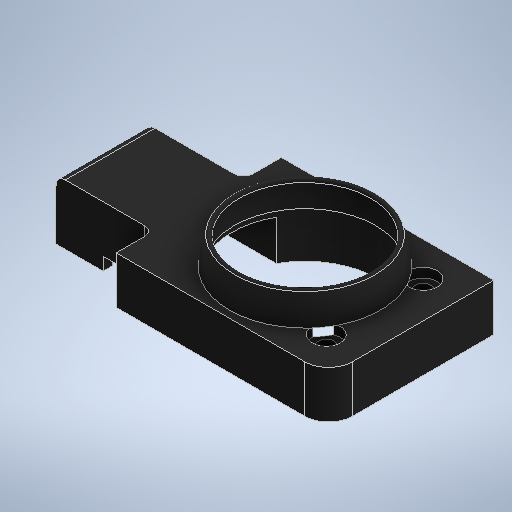
# Autodesk Inventor part: Joystick Shield
Saved by Autodesk Inventor 2025.4 (Build 294407000, 407)
## iProperties
Created: 2026-03-20
Part Number: Joystick Shield
Material: Generic
Document SubType Name: Modeling
Designer: lenovo
Density: 1 g/cm^3
Appearance: Default(1)
Author: lenovo
Autodesk Inventor part; units mm, degrees
ref_plane "YZ Plane" through (0, 0, 0) normal (1, 0, 0) x (0, 1, 0)
ref_plane "XZ Plane" through (0, 0, 0) normal (0, 1, 0) x (-1, 0, 0)
ref_plane "XY Plane" through (0, 0, 0) normal (0, 0, 1) x (1, 0, 0)
sketch "Sketch1" plane through (0, 0, 0) normal (0, 0, 1) x (1, 0, 0)
  line L0 (-22.5, -5) -> (22.5, -5)
  line L1 (22.5, -5) -> (22.5, 5)
  line L2 (22.5, 5) -> (-22.5, 5)
  line L3 (-22.5, 5) -> (-22.5, -5)
  line L4 (-22.5, -5) -> (22.5, 5) construction
  line L5 (22.5, -5) -> (-22.5, 5) construction
  point P0 (0, 0)
  dimension "d0" = 45
  dimension "d1" = 10
  constraints: 12 end point, 2 midpoint, 2 parallel, 1 horizontal, 1 perpendicular
  measures "d0" distance of L2.end L1.end
  measures "d1" distance of L2.end L0.start
extrude "Extrusion1" add sketch "Sketch1" along normal mid plane 35
sketch "Sketch2" plane through (0, 0, 0) normal (0, 0, 1) x (1, 0, 0)
  arc A0 (15, 5) -> (13.65, 11.2191) centre (0, 5) ccw
  line L0 (22.5, 5) -> (-22.5, 5) projected
  arc A1 (16, 5) -> (14.7419, 11.2191) centre (0, 5) ccw
  line L1 (13.65, 11.2191) -> (14.7419, 11.2191)
  line L2 (-22.5, -5) -> (22.5, -5) projected
  line L3 (0, -5) -> (0, 5)
  point P0 (0, 0)
  dimension "d4" = 15
  dimension "d6" = 1
  dimension "d24" = 27.3
  constraints: 4 end point, 4 point on circle, 3 midpoint, 2 centre point, 2 point on line, 1 coincident, 1 horizontal, 1 perpendicular
  measures "d4" radius of A0
  measures "d6" radial gap between concentric circles of A0 A1
  measures "d24" diameter of L1.start L3
revolve "Revolution1" add sketch "Sketch2" angle 360 about axis through (0, -5, 0) along (0, 1, 0)
fillet "Fillet1" radius 0.5 2 edges at (-14.7419, 11.2191, 0) (-13.65, 11.2191, 0)
sketch "Sketch3" plane through (-22.5, -5, 17.5) normal (0, -1, 0) x (1, 0, 0)
  circle A0 centre (22.5, -17.5) radius 14.75
  line L0 (45, 0) -> (45, -35) projected
  line L1 (0, 0) -> (45, 0) projected
  circle A1 centre (22.5, -17.5) radius 15 projected
  point P0 (45, -17.5)
  point P1 (22.5, 0)
  dimension "d9" = 29.5
  constraints: 2 midpoint, 1 centre point, 1 coincident, 1 concentric
  measures "d9" diameter of A0
extrude "Extrusion2" cut sketch "Sketch3" against normal up to surface (10 mm away) contours A0
sketch "Sketch4" plane through (-22.5, 5, 17.5) normal (0, 1, 0) x (1, 0, 0)
  circle A0 centre (37.25, 27.75) radius 1.65
  line L0 (45, 35) -> (45, 0) projected
  line L1 (0, 35) -> (45, 35) projected
  point P0 (22.5, 17.5)
  dimension "d12" = 3.3
  dimension "d13" = 7.75
  dimension "d14" = 7.25
  constraints: 1 centre point
  measures "d12" diameter of A0
  measures "d13" distance from line of L0 A0.centre
  measures "d14" distance from line of L1 A0.centre
extrude "Extrusion3" cut sketch "Sketch4" against normal blind 10
pattern_linear "Rectangular Pattern1" count 2 spacing 20.5 along (0, 0, 1) of "Extrusion3"
sketch "Sketch6" plane through (-22.5, -5, 17.5) normal (-1, 0, 0) x (0, 0, 1)
  line L0 (-10, 0) -> (-25, 0)
  line L1 (-25, 0) -> (-25, 8.5)
  line L2 (-25, 8.5) -> (-10, 8.5)
  line L3 (-10, 8.5) -> (-10, 0)
  line L4 (-10, 0) -> (-25, 8.5) construction
  line L5 (-25, 0) -> (-10, 8.5) construction
  line L6 (-35, 10) -> (0, 10) projected
  line L7 (0, 10) -> (0, 0) projected
  line L8 (-35, 0) -> (0, 0) projected
  point P0 (-17.5, 5)
  point P1 (-17.5, 4.25)
  point P2 (-17.5, 10)
  point P3 (-17.5, 0)
  dimension "d33" = 1.5
  dimension "d38" = 15
  constraints: 12 end point, 5 midpoint, 2 parallel, 1 horizontal, 1 perpendicular, 1 vertical alignment
  measures "d33" distance between parallel lines of L2 L6
  measures "d38" distance of L0.start L0.end
extrude "Extrusion5" cut sketch "Sketch6" against normal blind 15
sketch "Sketch8" plane through (-22.5, -5, -17.5) normal (0, -1, 0) x (1, 0, 0)
  circle A0 centre (22.5, 17.5) radius 15.5
  arc A1 (9.7991, 10) -> (9.7991, 25) centre (22.5, 17.5) ccw projected
  dimension "d39" = 31
  constraints: 1 centre point, 1 concentric
  measures "d39" diameter of A0
extrude "Extrusion6" cut sketch "Sketch8" against normal up to surface (10 mm away)
sketch "Sketch10" plane through (0, 0, 0) normal (0, 0, 1) x (1, 0, 0)
  line L0 (-22.5, -0.75) -> (-37.5, -0.75)
  line L1 (-37.5, -0.75) -> (-37.5, -7.75)
  line L2 (-22.5, 3.5) -> (-22.5, -5) projected
  point P0 (0, 0)
  dimension "d42" = 15
  dimension "d43" = 7
  constraints: 4 end point, 1 horizontal, 1 midpoint, 1 perpendicular
  measures "d42" distance of L0.start L0.end
  measures "d43" distance of L0.end L1.end
sketch "Sketch11" plane through (-22.5, -5, 17.5) normal (-1, 0, 0) x (0, 0, 1)
  line L0 (-27, 0) -> (-8, 0)
  line L1 (-8, 0) -> (-8, 10)
  line L2 (-8, 10) -> (-27, 10)
  line L3 (-27, 10) -> (-27, 0)
  line L4 (-27, 0) -> (-8, 10) construction
  line L5 (-8, 0) -> (-27, 10) construction
  line L6 (-35, 10) -> (0, 10) projected
  line L7 (-25, 8.5) -> (-10, 8.5) projected
  line L8 (-2, 0) -> (-33, 0) projected
  line L9 (-10, 8.5) -> (-10, 0) projected
  line L10 (-25, 0) -> (-25, 8.5) projected
  line L11 (-25, 0) -> (-25, 8.5)
  line L12 (-25, 8.5) -> (-10, 8.5)
  line L13 (-10, 0) -> (-8, 0)
  line L14 (-27, 0) -> (-25, 0)
  point P0 (-17.5, 5)
  point P1 (-17.5, 5)
  point P2 (-17.5, 10)
  point P3 (-17.5, 10)
  point P4 (-17.5, 8.5)
  point P5 (-17.5, 0)
  point P6 (-8, 5)
  point P7 (-10, 0)
  dimension "d44" = 2
  constraints: 20 end point, 9 midpoint, 3 parallel, 2 collinear, 2 perpendicular, 1 horizontal, 1 vertical alignment
  measures "d44" distance from line of point (-8, 5) L9
sweep "Sweep1" add profiles "Sketch11" path "Sketch10" path curves L0 L1 contours L3 L2 L1 L0 L9 L7 L10
fillet "Fillet2" radius 2 3 edges at (-43.25, 5, 0) (-22.5, 0, 9.5) (-22.5, 0, -9.5)
fillet "Fillet3" radius 5 1 edges at (22.5, 0, 17.5)
sketch "Sketch12" plane through (-22.5, 5, -17.5) normal (0, 1, 0) x (1, 0, 0)
  arc A0 (38.5, -17.5) -> (37.5, -17.5) centre (10.75, -27.75) ccw projected
  circle A1 centre (37.25, -27.75) radius 3
  circle A2 centre (37.25, -7.25) radius 3
  circle A3 centre (37.25, -27.75) radius 1.65 projected
  circle A4 centre (37.25, -7.25) radius 1.65 projected
  point P0 (22.5, -17.5)
  dimension "d51" = 6
  dimension "d52" = 6
  constraints: 2 centre point, 2 concentric, 1 other
  measures "d51" diameter of A1
  measures "d52" diameter of A2
extrude "Extrusion7" cut sketch "Sketch12" against normal blind 2 contours A1 | A2 | A3 | A4
body "Solid1"
